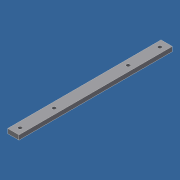
# Autodesk Inventor part: P1699_003_Support
Saved by Autodesk Inventor 2015 SP2 (Build 190223200, 223)
## iProperties
Created: 2017-01-26
Part Number: P1699_003_Support
Project: Nom Projet
Material: .
Description: Nom pièce
Document SubType Name: Modeling
Designer: Jean-Marc.VULLIAMY
Authority: brut Ø
Density: 1 g/cm^3
Appearance: Par défaut(1)
Material number: ---
Author: Jean-Marc.VULLIAMY
Autodesk Inventor part; units mm, degrees
ref_plane "Plan YZ" through (0, 0, 0) normal (1, 0, 0) x (0, 1, 0)
ref_plane "Plan XZ" through (0, 0, 0) normal (0, 1, 0) x (-1, 0, 0)
ref_plane "Plan XY" through (0, 0, 0) normal (0, 0, 1) x (1, 0, 0)
sketch "Esquisse7" plane through (0, 0, 0) normal (0, 0, 1) x (1, 0, 0)
  line L0 (-5, 68) -> (5, 68)
  line L1 (5, 68) -> (5, -68)
  line L2 (5, -68) -> (-5, -68)
  line L3 (-5, -68) -> (-5, 68)
  line L4 (0, 95.2) -> (0, -95.2) construction
  line L5 (-7, 0) -> (7, 0) construction
  point P0 (0, 0)
  point P1 (0, 62)
  point P2 (0, -62)
  point P3 (0, 33.92)
  point P4 (0, -31.73)
  dimension "d28" = 10
  dimension "d29" = 136
  dimension "d40" = 124
  dimension "d45" = 28.08
  dimension "d46" = 65.65
  dimension "d47" = 30.27
  constraints: 8 end point, 3 point on line, 2 parallel, 1 horizontal, 1 perpendicular, 1 symmetric about line, 2 other
  measures "d28" distance of L0.start L0.end
  measures "d29" distance of L2.end L0.start
  measures "d40" distance of point (0, -62) point (0, 62)
  measures "d45" distance of point (0, 33.92) point (0, 62)
  measures "d46" distance of point (0, -31.73) point (0, 33.92)
  measures "d47" distance of point (0, -62) point (0, -31.73)
extrude "Extrusion3" add sketch "Esquisse7" against normal blind 4
hole "Perçage3" at (0, 62, 0) at (0, -62, 0) at (0, 33.92, 0) at (0, -31.73, 0) direction (0, 0, -1) diameter 3.2 end through all
